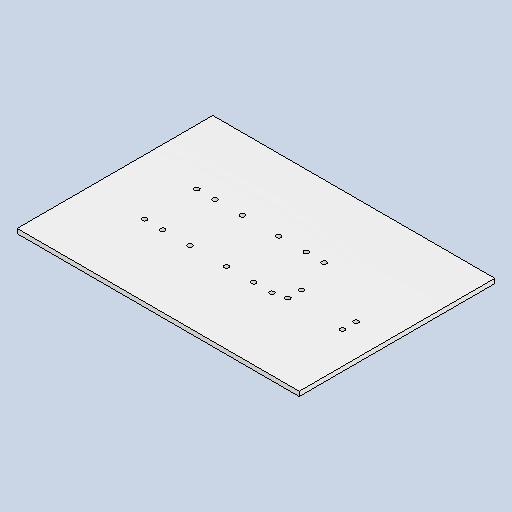
# Autodesk Inventor part: Mount PLate
Saved by Autodesk Inventor 2023.2 (Build 272271000, 271)
## iProperties
Created: 2024-01-25
Part Number: Mount PLate
Material: UHMW, White
Document SubType Name: Modeling
Designer: Nathan Cai
Density: 0.94 g/cm^3
Appearance: Smooth - White
Mass: 79.8087 g
Surface Area: 561.2 cm^2
Volume: 84.9029 cm^3
Author: Nathan Cai
Autodesk Inventor part; units mm, degrees
ref_plane "YZ Plane" through (0, 0, 0) normal (1, 0, 0) x (0, 1, 0)
ref_plane "XZ Plane" through (0, 0, 0) normal (0, 1, 0) x (-1, 0, 0)
ref_plane "XY Plane" through (0, 0, 0) normal (0, 0, 1) x (1, 0, 0)
sketch "Sketch1" plane through (0, 0, 0) normal (0, 1, 0) x (-1, 0, 0)
  line L0 (98.425, -68.2625) -> (-98.425, -68.2625)
  line L1 (-98.425, -68.2625) -> (-98.425, 68.2625)
  line L2 (-98.425, 68.2625) -> (98.425, 68.2625)
  line L3 (98.425, 68.2625) -> (98.425, -68.2625)
  line L4 (98.425, -68.2625) -> (-98.425, 68.2625) construction
  line L5 (-98.425, -68.2625) -> (98.425, 68.2625) construction
  point P0 (0, 0)
  point P1 (45.2437, 60.325)
  dimension "d11" = 136.525
  dimension "d13" = 196.85
  constraints: 12 end point, 2 midpoint, 2 parallel, 1 horizontal, 1 perpendicular
  measures "d11" distance of L0.end L1.end
  measures "d13" distance between parallel lines of L1 L3
extrude "Extrusion1" add sketch "Sketch1" along normal blind 3.175
sketch "Sketch2" plane through (0, 0, 0) normal (0, -1, 0) x (1, 0, 0)
  point P0 (76.2, 15.875)
  point P1 (29.3688, -18.2562)
  point P2 (16.6688, -18.2562)
  point P3 (29.3688, 18.2562)
  point P4 (16.6688, 18.2562)
  point P5 (-59.5312, 18.2562)
  point P6 (-46.8312, 18.2562)
  point P7 (-46.8312, -18.2562)
  point P8 (-59.5312, -18.2562)
  point P9 (-27.7812, 18.2562)
  point P10 (-2.3812, 18.2562)
  point P11 (-2.3812, -18.2562)
  point P12 (-27.7812, -18.2562)
  point P13 (76.2, 6.35)
  point P14 (38.1, 15.875)
  point P15 (38.1, 6.35)
hole "Hole1" at (76.2, 0, 15.875) at (29.3688, 0, -18.2562) at (16.6688, 0, -18.2562) at (29.3688, 0, 18.2562) at (16.6688, 0, 18.2562) at (-59.5312, 0, 18.2562) at (-46.8312, 0, 18.2562) at (-46.8312, 0, -18.2562) at (-59.5312, 0, -18.2562) at (-27.7812, 0, 18.2562) at (-2.3812, 0, 18.2562) at (-2.3812, 0, -18.2562) at (-27.7812, 0, -18.2562) at (76.2, 0, 6.35) at (38.1, 0, 15.875) at (38.1, 0, 6.35) direction (0, 1, 0) diameter 3.2639 end through all
body "Solid1"
